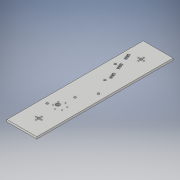
# Autodesk Inventor part: testPart_chassis9
Saved by Autodesk Inventor 2019 (Build 230136000, 136)
## iProperties
Created: 2019-09-17
Part Number: testPart_chassis9
Material: Generic
Document SubType Name: Modeling
Designer: shrey
Density: 1 g/cm^3
Appearance: Default
Author: shrey
Autodesk Inventor part; units mm, degrees
ref_plane "YZ Plane" through (0, 0, 0) normal (1, 0, 0) x (0, 1, 0)
ref_plane "XZ Plane" through (0, 0, 0) normal (0, 1, 0) x (-1, 0, 0)
ref_plane "XY Plane" through (0, 0, 0) normal (0, 0, 1) x (1, 0, 0)
sketch "Sketch1" plane through (0, 0, 0) normal (0, 1, 0) x (-1, 0, 0)
  line L0 (-44.45, -203.2) -> (44.45, -203.2)
  line L1 (44.45, -203.2) -> (44.45, 203.2)
  line L2 (44.45, 203.2) -> (-44.45, 203.2)
  line L3 (-44.45, 203.2) -> (-44.45, -203.2)
  line L4 (-44.45, -203.2) -> (44.45, 203.2) construction
  line L5 (44.45, -203.2) -> (-44.45, 203.2) construction
  line L6 (0, 203.2) -> (0, -203.2) construction
  line L7 (0, 0) -> (44.45, 0) construction
  line L8 (0, -203.2) -> (0, 203.2) construction
  line L9 (0, 152.4) -> (7.112, 152.4) construction
  line L10 (0, -152.4) -> (0, -203.2) construction
  circle A0 centre (0, -152.4) radius 4
  circle A1 centre (0, -152.4) radius 8 construction
  line L11 (0, 152.4) -> (-44.45, 152.4) construction
  line L12 (-44.45, 152.4) -> (-44.45, 88.9)
  line L13 (-44.45, 88.9) -> (0, 88.9) construction
  line L14 (0, 88.9) -> (0, 152.4) construction
  circle A2 centre (0, 88.9) radius 7.112 construction
  circle A3 centre (7.112, 88.9) radius 5.9944
  circle A4 centre (0, 88.9) radius 15.494 construction
  circle A5 centre (0, 104.394) radius 1.5
  circle A6 centre (0, 88.9) radius 15.494 construction
  circle A7 centre (-13.4182, 96.647) radius 1.5
  circle A8 centre (0, 88.9) radius 15.494 construction
  circle A9 centre (-13.4182, 81.153) radius 1.5
  circle A10 centre (0, 88.9) radius 15.494 construction
  circle A11 centre (0, 73.406) radius 1.5
  circle A12 centre (0, 88.9) radius 15.494 construction
  circle A13 centre (13.4182, 81.153) radius 1.5
  circle A14 centre (0, 88.9) radius 15.494 construction
  circle A15 centre (13.4182, 96.647) radius 1.5
  circle A16 centre (0, -144.4) radius 1.85
  circle A17 centre (-8, -152.4) radius 1.85
  circle A18 centre (0, -160.4) radius 1.85
  circle A19 centre (8, -152.4) radius 1.85
  circle A20 centre (0, 152.4) radius 4
  circle A21 centre (0, 152.4) radius 8 construction
  circle A22 centre (0, 160.4) radius 1.85
  circle A23 centre (0, 152.4) radius 8 construction
  circle A24 centre (-8, 152.4) radius 1.85
  circle A25 centre (0, 152.4) radius 8 construction
  circle A26 centre (0, 144.4) radius 1.85
  circle A27 centre (0, 152.4) radius 8 construction
  circle A28 centre (8, 152.4) radius 1.85
  line L15 (-88.9, 44.45) -> (0, 44.45) construction
  line L16 (0, 44.45) -> (0, -44.45) construction
  line L17 (0, -44.45) -> (-88.9, -44.45) construction
  line L18 (-88.9, -44.45) -> (-88.9, 44.45) construction
  line L19 (-88.9, 44.45) -> (0, -44.45) construction
  line L20 (0, 44.45) -> (-88.9, -44.45) construction
  circle A29 centre (0, 44.45) radius 2.9766
  circle A30 centre (0, -44.45) radius 2.9766
  line L21 (44.45, -203.2) -> (25.4, -203.2)
  line L22 (25.4, -203.2) -> (25.4, -101.6) construction
  line L23 (25.4, -101.6) -> (44.45, -101.6) construction
  line L24 (44.45, -101.6) -> (44.45, -203.2)
  circle A31 centre (25.9021, -101.6) radius 3.175
  circle A32 centre (25.9021, 101.6) radius 3.175
  line L25 (-44.45, -17.5714) -> (-25.4, -17.5714) construction
  line L26 (-25.4, -17.5714) -> (-25.4, 31.4423) construction
  line L27 (-25.4, 31.4423) -> (-44.45, 31.4423) construction
  line L28 (-44.45, 31.4423) -> (-44.45, -17.5714)
  circle A33 centre (-25.4, 0) radius 3.175
  line L29 (-44.45, -203.2) -> (0, -203.2)
  line L30 (-44.45, 0) -> (-44.45, -203.2)
  line L31 (-44.45, -203.2) -> (19.05, -203.2)
  line L32 (19.05, -203.2) -> (19.05, -25.4) construction
  line L33 (19.05, -25.4) -> (-44.45, -25.4) construction
  line L34 (-44.45, -25.4) -> (-44.45, -203.2)
  line L35 (44.45, -203.2) -> (48.4188, -203.2)
  line L36 (48.4188, -203.2) -> (48.4188, -176.8615) construction
  line L37 (48.4188, -176.8615) -> (44.45, -176.8615) construction
  line L38 (44.45, -176.8615) -> (44.45, -203.2)
  circle A34 centre (0, -44.45) radius 12.065 construction
  line L39 (-12.065, -44.45) -> (48.4188, -203.2) construction
  line L40 (-6.5005, -59.055) -> (0.282, -76.8567)
  line L41 (0.282, -76.8567) -> (6.2159, -74.5959)
  line L42 (6.2159, -74.5959) -> (-0.5666, -56.7942)
  line L43 (-0.5666, -56.7942) -> (-6.5005, -59.055)
  line L44 (13.8469, -112.4601) -> (19.7808, -110.1993)
  line L45 (19.7808, -110.1993) -> (12.9983, -92.3976)
  line L46 (12.9983, -92.3976) -> (7.0644, -94.6584)
  line L47 (7.0644, -94.6584) -> (13.8469, -112.4601)
  line L48 (27.4118, -148.0635) -> (33.3457, -145.8027)
  line L49 (33.3457, -145.8027) -> (26.5632, -128.001)
  line L50 (26.5632, -128.001) -> (20.6293, -130.2618)
  line L51 (20.6293, -130.2618) -> (27.4118, -148.0635)
  dimension "d17" = 16
  dimension "d26" = 14.224
  dimension "d28" = 30.988
  dimension "d40" = 16
  dimension "d98" = 24.13
  dimension "d0" = 406.4
  dimension "d1" = 88.9
  dimension "d2" = 152.4
  dimension "d16" = 8
  dimension "d24" = 44.45
  dimension "d25" = 63.5
  dimension "d27" = 11.9888
  dimension "d29" = 3
  dimension "d32" = 360
  dimension "d34" = 3.7
  dimension "d37" = 360
  dimension "d39" = 8
  dimension "d41" = 3.7
  dimension "d44" = 360
  dimension "d63" = 88.9
  dimension "d64" = 5.9531
  dimension "d65" = 5.9531
  dimension "d71" = 101.6
  dimension "d72" = 19.05
  dimension "d73" = 6.35
  dimension "d74" = 19.05
  dimension "d75" = 6.35
  dimension "d81" = 177.8
  dimension "d82" = 63.5
  dimension "d97" = 3.9688
  dimension "d105" = 19.05
  dimension "d106" = 6.35
  dimension "d109" = 38.1
  constraints: 104 end point, 22 centre point, 16 parallel, 12 coincident, 11 point on line, 9 horizontal, 8 perpendicular, 5 midpoint, 5 vertical alignment, 4 horizontal alignment, 4 symmetric about line, 1 collinear, 97 other
  measures "d0" distance of L0.end L1.end
  measures "d1" distance of L1.end L2.end
  measures "d2" distance of L7.start point (0, 152.4)
  measures "d16" diameter of A0
  measures "d24" distance of L9.start L11.end
  measures "d25" distance of L11.end L12.end
  measures "d27" diameter of A3
  measures "d29" diameter of A5
  measures "d34" diameter of A16
  measures "d39" diameter of A20
  measures "d41" diameter of A22
  measures "d63" distance of L17.end L15.start
  measures "d64" diameter of A29
  measures "d65" diameter of A30
  measures "d71" distance of L21.end L22.end
  measures "d72" distance of L22.end L23.end
  measures "d73" diameter of A31
  measures "d74" distance of L25.start L25.end
  measures "d75" diameter of A33
  measures "d81" distance of L31.end L32.end
  measures "d82" distance of L32.end L33.end
  measures "d97" distance of L0.end L35.end
  measures "d105" distance of L40.start L40.end
  measures "d106" distance of L41.end L40.end
  measures "d109" distance of L40.end L44.start
extrude "Extrusion9" add sketch "Sketch1" along normal blind 6.35
body "Solid9"
